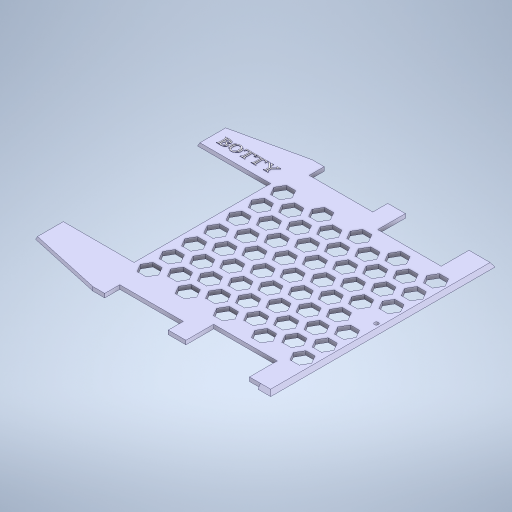
# Autodesk Inventor part: Bot v2 Top
Saved by Autodesk Inventor 2024 (Build 280153000, 153)
## iProperties
Created: 2023-11-01
Part Number: Bot v2 Top
Material: ABS Plastic
Document SubType Name: Modeling
Designer: CJ110
Density: 1.06 g/cm^3
Appearance: Smooth - White
Mass: 94.8046 g
Surface Area: 600.275 cm^2
Volume: 89.4383 cm^3
Author: CJ110
## iProperties of the stored document Bot v2 Top_3DPrint.ipt
Created: 2023-11-11
Part Number: Bot v2 Top_3DPrint
Material: Generic
Document SubType Name: Modeling
Designer: CJ110
Density: 1 g/cm^3
Appearance: Default
Author: CJ110
Autodesk Inventor part; units mm, degrees
(part 1 of 2)
ref_plane "YZ Plane" through (0, 0, 0) normal (1, 0, 0) x (0, 1, 0)
ref_plane "XZ Plane" through (0, 0, 0) normal (0, 1, 0) x (-1, 0, 0)
sketch "Sketch1" plane through (0, 0, 0) normal (0, 1, 0) x (-1, 0, 0)
  line L0 (0, 0) -> (144.1069, 0)
  line L1 (144.1069, 176.6621) -> (0, 176.6621)
  line L2 (0, 176.6621) -> (0, 0)
  line L3 (201.4652, 142.306) -> (144.8841, 142.306)
  line L4 (144.8841, 142.306) -> (144.8841, 34.356)
  line L5 (144.8841, 34.356) -> (201.4652, 34.356)
  line L6 (201.4652, 88.331) -> (0, 88.331) construction
  line L7 (144.1069, 176.6621) -> (201.4652, 164.0459)
  line L8 (201.4652, 12.6162) -> (144.1069, 0)
  line L9 (201.4652, 12.6162) -> (201.4652, 34.356)
  line L10 (201.4652, 142.306) -> (201.4652, 164.0459)
  line L11 (144.2491, 33.721) -> (144.2491, 142.941)
  line L12 (144.2491, 142.941) -> (200.8302, 142.941)
  line L13 (200.8302, 142.941) -> (200.8302, 163.5354)
  line L14 (200.8302, 163.5354) -> (144.0379, 176.0271)
  line L15 (144.0379, 176.0271) -> (0.635, 176.0271)
  line L16 (0.635, 176.0271) -> (0.635, 0.635)
  line L17 (0.635, 0.635) -> (144.0379, 0.635)
  line L18 (144.0379, 0.635) -> (200.8302, 13.1267)
  line L19 (200.8302, 13.1267) -> (200.8302, 33.721)
  line L20 (200.8302, 33.721) -> (144.2491, 33.721)
  line L21 (0.635, 176.0271) -> (0, 176.0271)
  line L22 (0.635, 0.635) -> (0, 0.635)
  point P0 (144.8841, 88.331)
  dimension "d0" = 176.6621
  dimension "d2" = 56.581
  dimension "d3" = 107.95
  dimension "d10" = 21.7399
  dimension "d11" = 144.1069
  dimension "d12" = 21.7399
  dimension "d52" = 201.4652
  dimension "d53" = 144.1069
  dimension "d54" = 0.635
  constraints: 46 end point, 12 perpendicular, 6 parallel, 3 horizontal, 3 point on line, 2 collinear, 2 midpoint, 9 other
  measures "d0" distance of L1.end L0.start
  measures "d2" distance of L3.start L3.end
  measures "d3" distance of L3.end L4.end
  measures "d10" distance from line of L7.end L3
  measures "d11" distance from line of L0.end L2
  measures "d12" distance from line of L8.start L5
  measures "d52" distance between parallel lines of L2 L9
  measures "d53" distance from line of L2 L1.start
  measures "d54" distance between parallel lines of L4 L11
extrude "Extrusion1" add sketch "Sketch1" along normal blind 3.175 contours L2 L21 L16 L22 | L16 L15 L14 L13 L12 L11 L20 L19 L18 L17
chamfer "Chamfer1" [suppressed]
sketch "Sketch2" plane through (0, 0, 0) normal (0, -1, 0) x (1, 0, 0)
  line L0 (0, 176.0271) -> (0, 0.635) projected
  line L1 (-145.8366, 33.721) -> (-145.8366, 142.941)
  line L2 (-144.0379, 176.0271) -> (0, 176.0271) projected
  line L3 (-200.8302, 163.5354) -> (-144.0379, 176.0271) projected
  line L4 (-200.8302, 142.941) -> (-200.8302, 163.5354) projected
  line L5 (-144.2491, 142.941) -> (-200.8302, 142.941) projected
  line L6 (-144.2491, 33.721) -> (-144.2491, 142.941) projected
  line L7 (-200.8302, 33.721) -> (-144.2491, 33.721) projected
  line L8 (-200.8302, 13.1267) -> (-200.8302, 33.721) projected
  line L9 (-144.0379, 0.635) -> (-200.8302, 13.1267) projected
  line L10 (0, 0.635) -> (-144.0379, 0.635) projected
  point P0 (0, 0)
  dimension "d55" = 1.5875
  constraints: 2 end point, 2 point on line
  measures "d55" distance between parallel lines of L6 L1
extrude "Extrusion2" add sketch "Sketch2" against normal blind 1.5875 contours L5 L6 L7 L1
sketch "Sketch3" plane through (0, 0, 195.7121) normal (1, 0, 0) x (0, 0, -1)
  line L0 (195.7121, 20.32) -> (195.7121, 0)
  line L1 (195.7121, 20.32) -> (183.0121, 20.32)
  line L2 (183.0121, 20.32) -> (195.7121, 0)
  line L3 (19.685, 0) -> (195.0771, 0) projected
  line L4 (19.685, 3.175) -> (195.0771, 3.175) projected
  line L5 (0, 0) -> (12.7, 20.32)
  line L6 (12.7, 20.32) -> (0, 20.32)
  line L7 (0, 20.32) -> (0, 0)
  line L8 (195.0771, 0) -> (195.0771, 3.175) projected
  line L9 (19.685, 0) -> (19.685, 3.175) projected
  point P0 (195.7121, 3.175)
  point P1 (193.7277, 3.175)
  point P2 (1.9844, 3.175)
  point P3 (195.0771, 1.016)
  point P4 (0.635, 1.016)
  dimension "d18" = 20.32
  dimension "d19" = 12.7
  dimension "d20" = 20.32
  dimension "d21" = 12.7
  constraints: 12 end point, 2 coincident, 2 horizontal, 2 vertical, 1 horizontal alignment
  measures "d18" distance of L0.start L0.end
  measures "d19" distance of L0.start L1.end
  measures "d20" distance of L6.end L5.start
  measures "d21" distance of L5.end L6.end
extrude "Extrusion3" [suppressed]
sketch "Sketch4" plane through (-147.1066, 0, 142.941) normal (0, 0, -1) x (-1, 0, 0)
  line L0 (53.7235, 0) -> (60.0735, 0)
  line L1 (53.7235, 0) -> (53.7235, 10.16)
  line L2 (53.7235, 10.16) -> (60.0735, 0)
  line L3 (53.7235, 0) -> (53.7235, 3.175) projected
  line L4 (-3.0688, 0) -> (53.7235, 0) projected
  line L5 (53.7235, 3.175) -> (55.7079, 0)
  point P0 (-147.1066, 0)
  point P1 (53.7235, 3.175)
  dimension "d38" = 6.35
  dimension "d39" = 10.16
  constraints: 8 end point, 2 collinear, 1 horizontal, 1 parallel, 1 point on line, 1 vertical
  measures "d38" distance of L0.start L0.end
  measures "d39" distance of L0.start L1.end
extrude "Extrusion4" add sketch "Sketch4" against normal up to surface contours L1 L5 L0 surface through (-200.8302, 0, 163.5354) normal (-0.2148189, 0, 0.9766539)
sketch "Sketch5" plane through (0, 3.175, 0) normal (0, 1, 0) x (1, 0, 0)
  line L0 (-144.1069, 0) -> (-201.4652, -22.1412) projected
  line L1 (-172.786, -11.0706) -> (-139.2855, -97.856)
  line L2 (-139.2855, -97.856) -> (-172.786, -184.6415)
  line L3 (-201.4652, -173.5709) -> (-144.1069, -195.7121) projected
  point P0 (0, 0)
  point P1 (-149.5475, -1.9844)
  point P2 (-199.4808, -23.2787)
  point P3 (-199.4808, -176.4009)
  point P4 (-149.5475, -197.6952)
  point P5 (-201.4652, -22.1412)
  point P6 (-144.1069, 0)
  point P7 (-146.116, -195.7121)
  constraints: 4 end point, 6 other
ref_plane "Work Plane1" through (-139.2855, 3.175, 97.856) normal (-0.9329073, 0, -0.3601166) x (-0.3601166, 0, 0.9329073)
ref_plane "Work Plane2" through (-172.786, 3.175, 11.0706) normal (-0.9329073, 0, 0.3601166) x (0.3601166, 0, 0.9329073)
sketch "Sketch6" plane through (-139.2855, 3.175, 97.856) normal (-0.9329073, 0, -0.3601166) x (-0.3601166, 0, 0.9329073)
  line L0 (82.1072, 17.145) -> (94.8072, -3.175)
  line L1 (94.8072, -3.175) -> (94.8072, 17.145)
  line L2 (94.8072, 17.145) -> (82.1072, 17.145)
  point P0 (-141.4496, -3.175)
  dimension "d30" = 12.7
  dimension "d31" = 20.32
  constraints: 6 end point, 1 coincident, 1 perpendicular, 1 vertical
  measures "d30" distance of L1.end L0.start
  measures "d31" distance of L0.end L1.end
extrude "Extrusion5" [suppressed]
sketch "Sketch7" plane through (-172.786, 3.175, 11.0706) normal (-0.9329073, 0, 0.3601166) x (0.3601166, 0, 0.9329073)
  line L0 (12.7, 17.145) -> (0, -3.175)
  line L1 (0, -3.175) -> (0, 17.145)
  line L2 (0, 17.145) -> (12.7, 17.145)
  point P0 (51.8953, -3.175)
  point P1 (0, -3.175)
  dimension "d34" = 12.7
  dimension "d35" = 20.32
  constraints: 6 end point, 1 coincident, 1 perpendicular, 1 vertical
  measures "d34" distance of L1.end L0.start
  measures "d35" distance of L0.end L1.end
extrude "Extrusion6" [suppressed]
ref_plane "Work Plane3" through (-144.2491, 1.5875, 88.331) normal (0, 0, -1) x (-1, 0, 0)
mirror "Mirror1" about plane through (-144.2491, 1.5875, 88.331) normal (0, 0, -1) of "Extrusion4"
sketch "Sketch8" plane through (0, 0, 176.6621) normal (1, 0, 0) x (0, 0, -1)
  line L0 (0.635, 0) -> (13.5632, 0) projected
  line L1 (0.635, 0) -> (-5.715, 0)
  line L2 (0.635, 0) -> (0.635, 10.16)
  line L3 (0.635, 10.16) -> (-5.715, 0)
  line L4 (0.635, 3.175) -> (-1.3494, 0)
  line L5 (0.635, 0) -> (0.635, 3.175) projected
  line L6 (0.635, 0) -> (176.0271, 0) projected
  line L7 (176.0271, 0) -> (176.0271, 3.175) projected
  line L8 (0.635, 3.175) -> (176.0271, 3.175) projected
  line L9 (0.635, 0) -> (0.635, 3.175) projected
  point P0 (176.6621, 0)
  point P1 (22.9072, 0)
  dimension "d40" = 6.35
  dimension "d41" = 10.16
  constraints: 8 end point, 2 collinear, 1 horizontal, 1 parallel, 1 point on line, 1 vertical
  measures "d40" distance of L0.start L1.end
  measures "d41" distance of L0.start L2.end
extrude "Extrusion7" add sketch "Sketch8" against normal blind 10.16 contours L1 L4 L2
mirror "Mirror2" about plane through (-144.2491, 1.5875, 88.331) normal (0, 0, -1) of "Extrusion7"
sketch "Sketch9" plane through (0, 3.175, 0) normal (0, 1, 0) x (1, 0, 0)
  line L0 (-69.6824, -175.4708) -> (-18.8824, -175.4708)
  line L1 (-18.8824, -175.4708) -> (-18.8824, -153.8808)
  line L2 (-18.8824, -153.8808) -> (-69.6824, -153.8808)
  line L3 (-69.6824, -153.8808) -> (-69.6824, -175.4708)
  line L4 (-134.5971, -175.4708) -> (-83.7971, -175.4708)
  line L5 (-83.7971, -175.4708) -> (-83.7971, -164.0408)
  line L6 (-83.7971, -164.0408) -> (-134.5971, -164.0408)
  line L7 (-134.5971, -164.0408) -> (-134.5971, -175.4708)
  line L8 (-144.2491, -33.721) -> (-144.2491, -142.941) projected
  line L9 (-144.2491, -88.331) -> (0, -88.331) construction
  line L10 (0, -176.0271) -> (0, -0.635) projected
  line L11 (-145.8366, -33.721) -> (-145.8366, -142.941) projected
  line L12 (-69.6824, -1.1913) -> (-18.8824, -1.1913)
  line L13 (-18.8824, -0.635) -> (-18.8824, -22.7813)
  line L14 (-18.8824, -22.7813) -> (-69.6824, -22.7813)
  line L15 (-69.6824, -22.7813) -> (-69.6824, -0.635)
  line L16 (-134.5971, -1.1913) -> (-83.7971, -1.1913)
  line L17 (-83.7971, -0.635) -> (-83.7971, -12.6213)
  line L18 (-83.7971, -12.6213) -> (-134.5971, -12.6213)
  line L19 (-134.5971, -12.6213) -> (-134.5971, -0.635)
  line L20 (0, -0.635) -> (0, -176.0271)
  line L21 (-69.6824, -175.4708) -> (-69.6824, -176.0271)
  line L22 (-144.0379, -176.0271) -> (-10.16, -176.0271) projected
  line L23 (-18.8824, -175.4708) -> (-18.8824, -176.0271)
  line L24 (-83.7971, -175.4708) -> (-83.7971, -176.0271)
  line L25 (-134.5971, -175.4708) -> (-134.5971, -176.0271)
  line L26 (0, -176.0271) -> (0, -0.635) projected
  line L27 (0, -0.635) -> (-10.16, -0.635) projected
  line L28 (-10.16, -0.635) -> (-144.0379, -0.635) projected
  line L29 (-144.0379, -0.635) -> (-200.8302, -13.1267) projected
  line L30 (-200.8302, -13.1267) -> (-200.8302, -33.721) projected
  line L31 (-200.8302, -33.721) -> (-144.2491, -33.721) projected
  line L32 (-144.2491, -33.721) -> (-144.2491, -142.941) projected
  line L33 (-144.2491, -142.941) -> (-200.8302, -142.941) projected
  line L34 (-200.8302, -142.941) -> (-200.8302, -163.5354) projected
  line L35 (-200.8302, -163.5354) -> (-144.0379, -176.0271) projected
  line L36 (-144.0379, -176.0271) -> (-10.16, -176.0271) projected
  line L37 (-10.16, -176.0271) -> (0, -176.0271) projected
  point P0 (0, 0)
  point P1 (-44.2824, -153.8808)
  point P2 (-109.1971, -164.0408)
  point P3 (-44.2824, -22.7813)
  point P4 (-109.1971, -12.6213)
  point P5 (-83.7971, -176.0271)
  point P6 (-18.8824, -176.0271)
  dimension "d44" = 11.43
  dimension "d45" = 21.59
  dimension "d60" = 65.5498
  dimension "d61" = 50.8
  dimension "d62" = 50.8
  dimension "d63" = 64.9148
  dimension "d69" = 9.652
  constraints: 44 end point, 14 point on line, 12 symmetric about line, 5 perpendicular, 4 midpoint, 4 parallel, 2 horizontal, 1 vertical
  measures "d44" distance between parallel lines of L6 L4
  measures "d45" distance between parallel lines of L2 L0
  measures "d60" distance between parallel lines of L9 L2
  measures "d61" distance between parallel lines of L7 L5
  measures "d62" distance of L1.end L2.end
  measures "d63" horizontal distance of point (-44.282, -153.881) point (-109.197, -164.041)
  measures "d69" distance between parallel lines of L7 L8
sketch "Sketch11" plane through (-144.2491, 1.5875, 88.331) normal (0, 0, -1) x (-1, 0, 0)
  line L0 (-144.2491, 1.5875) -> (-144.2491, -1.5875) projected
  line L1 (-144.2491, -1.5875) -> (-150.5991, -1.5875)
  line L2 (-150.5991, -1.5875) -> (-144.2491, 8.5725)
  line L3 (-144.2491, 8.5725) -> (-144.2491, -1.5875)
  line L4 (-144.2491, -1.5875) -> (-142.2648, 1.5875)
  line L5 (-134.0891, 1.5875) -> (-144.2491, 1.5875) projected
  dimension "d56" = 6.35
  dimension "d57" = 10.16
  constraints: 8 end point, 1 horizontal, 1 parallel, 1 perpendicular, 1 point on line
  measures "d56" distance of L0.end L1.end
  measures "d57" distance of L2.end L0.end
extrude "Extrusion9" cut sketch "Sketch11" along normal through all both and the other way through all contours L5 L4 L0
extrude "Extrusion10" cut sketch "Sketch9" against normal through all contours L3 L2 L1 L0 | L0 L23 L22 L21 | L22 L25 L4 L24 | L4 L7 L6 L5 | L13 L12 L15 L28 | L13 L14 L15 L12 | L17 L16 L19 L28 | L17 L18 L19 L16
sketch "Sketch12" plane through (0, 3.175, 0) normal (0, 1, 0) x (1, 0, 0)
  line L0 (-1.9844, -176.0271) -> (-1.9844, -0.635) projected
  line L1 (-1.9844, -88.331) -> (-144.2491, -88.331) construction
  line L2 (-144.2491, -33.721) -> (-144.2491, -142.941) projected
  circle A0 centre (-5.1594, -88.331) radius 1.5875
  point P0 (0, 0)
  dimension "d70" = 3.175
  dimension "d71" = 3.175
  constraints: 2 end point, 2 midpoint, 1 centre point, 1 point on line
  measures "d70" diameter of A0
  measures "d71" distance from line of L0 A0.centre
extrude "Extrusion11" cut sketch "Sketch12" against normal through all
sketch "Sketch16" plane through (0, 3.175, 0) normal (0, 1, 0) x (1, 0, 0)
  line L0 (-140.4391, -141.671) -> (-136.773, -135.321)
  line L1 (-136.773, -135.321) -> (-129.4406, -135.321)
  line L2 (-129.4406, -135.321) -> (-125.7744, -141.671)
  line L3 (-125.7744, -141.671) -> (-129.4406, -148.021)
  line L4 (-129.4406, -148.021) -> (-136.773, -148.021)
  line L5 (-136.773, -148.021) -> (-140.4391, -141.671)
  line L6 (-125.0412, -132.781) -> (-121.375, -126.431)
  line L7 (-121.375, -126.431) -> (-114.0427, -126.431)
  line L8 (-114.0427, -126.431) -> (-110.3765, -132.781)
  line L9 (-110.3765, -132.781) -> (-114.0427, -139.131)
  line L10 (-114.0427, -139.131) -> (-121.375, -139.131)
  line L11 (-121.375, -139.131) -> (-125.0412, -132.781)
  line L12 (-140.4391, -123.891) -> (-136.773, -117.541)
  line L13 (-136.773, -117.541) -> (-129.4406, -117.541)
  line L14 (-129.4406, -117.541) -> (-125.7744, -123.891)
  line L15 (-125.7744, -123.891) -> (-129.4406, -130.241)
  line L16 (-129.4406, -130.241) -> (-136.773, -130.241)
  line L17 (-136.773, -130.241) -> (-140.4391, -123.891)
  line L18 (-125.0412, -115.001) -> (-121.375, -108.651)
  line L19 (-121.375, -108.651) -> (-114.0427, -108.651)
  line L20 (-114.0427, -108.651) -> (-110.3765, -115.001)
  line L21 (-110.3765, -115.001) -> (-114.0427, -121.351)
  line L22 (-114.0427, -121.351) -> (-121.375, -121.351)
  line L23 (-121.375, -121.351) -> (-125.0412, -115.001)
  circle A0 centre (-5.1594, -97.856) radius 1.5875 projected
  line L24 (-69.6824, -22.7813) -> (-69.6824, -0.635) projected
  line L25 (-69.6824, -0.635) -> (-83.7971, -0.635) projected
  line L26 (-83.7971, -0.635) -> (-83.7971, -12.6213) projected
  line L27 (-83.7971, -12.6213) -> (-134.5971, -12.6213) projected
  line L28 (-134.5971, -12.6213) -> (-134.5971, -0.635) projected
  line L29 (-134.5971, -0.635) -> (-143.9886, -0.635) projected
  line L30 (-143.9886, -0.635) -> (-200.8302, -22.5767) projected
  line L31 (-200.8302, -22.5767) -> (-200.8302, -43.246) projected
  line L32 (-200.8302, -43.246) -> (-144.2491, -43.246) projected
  line L33 (-144.2491, -43.246) -> (-144.2491, -152.466) projected
  line L34 (-144.2491, -152.466) -> (-200.8302, -152.466) projected
  line L35 (-200.8302, -152.466) -> (-200.8302, -173.1354) projected
  line L36 (-200.8302, -173.1354) -> (-143.9886, -195.0771) projected
  line L37 (-143.9886, -195.0771) -> (-134.5971, -195.0771) projected
  line L38 (-134.5971, -195.0771) -> (-134.5971, -183.0908) projected
  line L39 (-134.5971, -183.0908) -> (-83.7971, -183.0908) projected
  line L40 (-83.7971, -183.0908) -> (-83.7971, -195.0771) projected
  line L41 (-83.7971, -195.0771) -> (-69.6824, -195.0771) projected
  line L42 (-69.6824, -195.0771) -> (-69.6824, -172.9308) projected
  line L43 (-69.6824, -172.9308) -> (-18.8824, -172.9308) projected
  line L44 (-18.8824, -172.9308) -> (-18.8824, -195.0771) projected
  line L45 (-18.8824, -195.0771) -> (-10.16, -195.0771) projected
  line L46 (-10.16, -195.0771) -> (-1.9844, -195.0771) projected
  line L47 (-1.9844, -195.0771) -> (-1.9844, -0.635) projected
  line L48 (-1.9844, -0.635) -> (-10.16, -0.635) projected
  line L49 (-10.16, -0.635) -> (-18.8824, -0.635) projected
  line L50 (-18.8824, -0.635) -> (-18.8824, -22.7813) projected
  line L51 (-18.8824, -22.7813) -> (-69.6824, -22.7813) projected
  line L52 (-110.3765, -97.221) -> (-114.0427, -103.571)
  line L53 (-114.0427, -73.091) -> (-110.3765, -79.441)
  line L54 (-114.0427, -90.871) -> (-110.3765, -97.221)
  line L55 (-125.7744, -106.111) -> (-129.4406, -112.461)
  line L56 (-129.4406, -99.761) -> (-125.7744, -106.111)
  line L57 (-121.375, -73.091) -> (-114.0427, -73.091)
  line L58 (-129.4406, -112.461) -> (-136.773, -112.461)
  line L59 (-136.773, -112.461) -> (-140.4391, -106.111)
  line L60 (-125.0412, -79.441) -> (-121.375, -73.091)
  line L61 (-140.4391, -106.111) -> (-136.773, -99.761)
  line L62 (-121.375, -103.571) -> (-125.0412, -97.221)
  line L63 (-114.0427, -103.571) -> (-121.375, -103.571)
  line L64 (-125.0412, -97.221) -> (-121.375, -90.871)
  line L65 (-121.375, -90.871) -> (-114.0427, -90.871)
  line L66 (-136.773, -99.761) -> (-129.4406, -99.761)
  line L67 (-114.0427, -85.791) -> (-121.375, -85.791)
  line L68 (-110.3765, -79.441) -> (-114.0427, -85.791)
  line L69 (-121.375, -85.791) -> (-125.0412, -79.441)
  line L70 (-129.4406, -94.681) -> (-136.773, -94.681)
  line L71 (-129.4406, -81.981) -> (-125.7744, -88.331)
  line L72 (-136.773, -94.681) -> (-140.4391, -88.331)
  line L73 (-136.773, -81.981) -> (-129.4406, -81.981)
  line L74 (-140.4391, -88.331) -> (-136.773, -81.981)
  line L75 (-125.7744, -88.331) -> (-129.4406, -94.681)
  line L76 (-110.3765, -61.661) -> (-114.0427, -68.011)
  line L77 (-114.0427, -37.531) -> (-110.3765, -43.881)
  line L78 (-114.0427, -55.311) -> (-110.3765, -61.661)
  line L79 (-125.7744, -70.551) -> (-129.4406, -76.901)
  line L80 (-129.4406, -64.201) -> (-125.7744, -70.551)
  line L81 (-121.375, -37.531) -> (-114.0427, -37.531)
  line L82 (-129.4406, -76.901) -> (-136.773, -76.901)
  line L83 (-136.773, -76.901) -> (-140.4391, -70.551)
  line L84 (-125.0412, -43.881) -> (-121.375, -37.531)
  line L85 (-140.4391, -70.551) -> (-136.773, -64.201)
  line L86 (-121.375, -68.011) -> (-125.0412, -61.661)
  line L87 (-114.0427, -68.011) -> (-121.375, -68.011)
  line L88 (-125.0412, -61.661) -> (-121.375, -55.311)
  line L89 (-121.375, -55.311) -> (-114.0427, -55.311)
  line L90 (-136.773, -64.201) -> (-129.4406, -64.201)
  line L91 (-114.0427, -50.231) -> (-121.375, -50.231)
  line L92 (-110.3765, -43.881) -> (-114.0427, -50.231)
  line L93 (-121.375, -50.231) -> (-125.0412, -43.881)
  line L94 (-129.4406, -59.121) -> (-136.773, -59.121)
  line L95 (-129.4406, -46.421) -> (-125.7744, -52.771)
  line L96 (-136.773, -59.121) -> (-140.4391, -52.771)
  line L97 (-136.773, -46.421) -> (-129.4406, -46.421)
  line L98 (-140.4391, -52.771) -> (-136.773, -46.421)
  line L99 (-125.7744, -52.771) -> (-129.4406, -59.121)
  line L100 (-79.8965, -132.781) -> (-83.5627, -139.131)
  line L101 (-83.5627, -108.651) -> (-79.8965, -115.001)
  line L102 (-83.5627, -126.431) -> (-79.8965, -132.781)
  line L103 (-95.2944, -141.671) -> (-98.9606, -148.021)
  line L104 (-98.9606, -135.321) -> (-95.2944, -141.671)
  line L105 (-90.895, -108.651) -> (-83.5627, -108.651)
  line L106 (-98.9606, -148.021) -> (-106.293, -148.021)
  line L107 (-106.293, -148.021) -> (-109.9591, -141.671)
  line L108 (-94.5612, -115.001) -> (-90.895, -108.651)
  line L109 (-109.9591, -141.671) -> (-106.293, -135.321)
  line L110 (-90.895, -139.131) -> (-94.5612, -132.781)
  line L111 (-83.5627, -139.131) -> (-90.895, -139.131)
  line L112 (-94.5612, -132.781) -> (-90.895, -126.431)
  line L113 (-90.895, -126.431) -> (-83.5627, -126.431)
  line L114 (-106.293, -135.321) -> (-98.9606, -135.321)
  line L115 (-83.5627, -121.351) -> (-90.895, -121.351)
  line L116 (-79.8965, -115.001) -> (-83.5627, -121.351)
  line L117 (-90.895, -121.351) -> (-94.5612, -115.001)
  line L118 (-98.9606, -130.241) -> (-106.293, -130.241)
  line L119 (-98.9606, -117.541) -> (-95.2944, -123.891)
  line L120 (-106.293, -130.241) -> (-109.9591, -123.891)
  line L121 (-106.293, -117.541) -> (-98.9606, -117.541)
  line L122 (-109.9591, -123.891) -> (-106.293, -117.541)
  line L123 (-95.2944, -123.891) -> (-98.9606, -130.241)
  line L124 (-79.8965, -97.221) -> (-83.5627, -103.571)
  line L125 (-83.5627, -73.091) -> (-79.8965, -79.441)
  line L126 (-83.5627, -90.871) -> (-79.8965, -97.221)
  line L127 (-95.2944, -106.111) -> (-98.9606, -112.461)
  line L128 (-98.9606, -99.761) -> (-95.2944, -106.111)
  line L129 (-90.895, -73.091) -> (-83.5627, -73.091)
  line L130 (-98.9606, -112.461) -> (-106.293, -112.461)
  line L131 (-106.293, -112.461) -> (-109.9591, -106.111)
  line L132 (-94.5612, -79.441) -> (-90.895, -73.091)
  line L133 (-109.9591, -106.111) -> (-106.293, -99.761)
  line L134 (-90.895, -103.571) -> (-94.5612, -97.221)
  line L135 (-83.5627, -103.571) -> (-90.895, -103.571)
  line L136 (-94.5612, -97.221) -> (-90.895, -90.871)
  line L137 (-90.895, -90.871) -> (-83.5627, -90.871)
  line L138 (-106.293, -99.761) -> (-98.9606, -99.761)
  line L139 (-83.5627, -85.791) -> (-90.895, -85.791)
  line L140 (-79.8965, -79.441) -> (-83.5627, -85.791)
  line L141 (-90.895, -85.791) -> (-94.5612, -79.441)
  line L142 (-98.9606, -94.681) -> (-106.293, -94.681)
  line L143 (-98.9606, -81.981) -> (-95.2944, -88.331)
  line L144 (-106.293, -94.681) -> (-109.9591, -88.331)
  line L145 (-106.293, -81.981) -> (-98.9606, -81.981)
  line L146 (-109.9591, -88.331) -> (-106.293, -81.981)
  line L147 (-95.2944, -88.331) -> (-98.9606, -94.681)
  line L148 (-79.8965, -61.661) -> (-83.5627, -68.011)
  line L149 (-83.5627, -37.531) -> (-79.8965, -43.881)
  line L150 (-83.5627, -55.311) -> (-79.8965, -61.661)
  line L151 (-95.2944, -70.551) -> (-98.9606, -76.901)
  line L152 (-98.9606, -64.201) -> (-95.2944, -70.551)
  line L153 (-90.895, -37.531) -> (-83.5627, -37.531)
  line L154 (-98.9606, -76.901) -> (-106.293, -76.901)
  line L155 (-106.293, -76.901) -> (-109.9591, -70.551)
  line L156 (-94.5612, -43.881) -> (-90.895, -37.531)
  line L157 (-109.9591, -70.551) -> (-106.293, -64.201)
  line L158 (-90.895, -68.011) -> (-94.5612, -61.661)
  line L159 (-83.5627, -68.011) -> (-90.895, -68.011)
  line L160 (-94.5612, -61.661) -> (-90.895, -55.311)
  line L161 (-90.895, -55.311) -> (-83.5627, -55.311)
  line L162 (-106.293, -64.201) -> (-98.9606, -64.201)
  line L163 (-83.5627, -50.231) -> (-90.895, -50.231)
  line L164 (-79.8965, -43.881) -> (-83.5627, -50.231)
  line L165 (-90.895, -50.231) -> (-94.5612, -43.881)
  line L166 (-98.9606, -59.121) -> (-106.293, -59.121)
  line L167 (-98.9606, -46.421) -> (-95.2944, -52.771)
  line L168 (-106.293, -59.121) -> (-109.9591, -52.771)
  line L169 (-106.293, -46.421) -> (-98.9606, -46.421)
  line L170 (-109.9591, -52.771) -> (-106.293, -46.421)
  line L171 (-95.2944, -52.771) -> (-98.9606, -59.121)
  line L172 (-49.4165, -132.781) -> (-53.0827, -139.131)
  line L173 (-53.0827, -108.651) -> (-49.4165, -115.001)
  line L174 (-53.0827, -126.431) -> (-49.4165, -132.781)
  line L175 (-64.8144, -141.671) -> (-68.4806, -148.021)
  line L176 (-68.4806, -135.321) -> (-64.8144, -141.671)
  line L177 (-60.415, -108.651) -> (-53.0827, -108.651)
  line L178 (-68.4806, -148.021) -> (-75.813, -148.021)
  line L179 (-75.813, -148.021) -> (-79.4791, -141.671)
  line L180 (-64.0812, -115.001) -> (-60.415, -108.651)
  line L181 (-79.4791, -141.671) -> (-75.813, -135.321)
  line L182 (-60.415, -139.131) -> (-64.0812, -132.781)
  line L183 (-53.0827, -139.131) -> (-60.415, -139.131)
  line L184 (-64.0812, -132.781) -> (-60.415, -126.431)
  line L185 (-60.415, -126.431) -> (-53.0827, -126.431)
  line L186 (-75.813, -135.321) -> (-68.4806, -135.321)
  line L187 (-53.0827, -121.351) -> (-60.415, -121.351)
  line L188 (-49.4165, -115.001) -> (-53.0827, -121.351)
  line L189 (-60.415, -121.351) -> (-64.0812, -115.001)
  line L190 (-68.4806, -130.241) -> (-75.813, -130.241)
  line L191 (-68.4806, -117.541) -> (-64.8144, -123.891)
  line L192 (-75.813, -130.241) -> (-79.4791, -123.891)
  line L193 (-75.813, -117.541) -> (-68.4806, -117.541)
  line L194 (-79.4791, -123.891) -> (-75.813, -117.541)
  line L195 (-64.8144, -123.891) -> (-68.4806, -130.241)
  line L196 (-49.4165, -97.221) -> (-53.0827, -103.571)
  line L197 (-53.0827, -73.091) -> (-49.4165, -79.441)
  line L198 (-53.0827, -90.871) -> (-49.4165, -97.221)
  line L199 (-64.8144, -106.111) -> (-68.4806, -112.461)
  line L200 (-68.4806, -99.761) -> (-64.8144, -106.111)
  line L201 (-60.415, -73.091) -> (-53.0827, -73.091)
  line L202 (-68.4806, -112.461) -> (-75.813, -112.461)
  line L203 (-75.813, -112.461) -> (-79.4791, -106.111)
  line L204 (-64.0812, -79.441) -> (-60.415, -73.091)
  line L205 (-79.4791, -106.111) -> (-75.813, -99.761)
  line L206 (-60.415, -103.571) -> (-64.0812, -97.221)
  line L207 (-53.0827, -103.571) -> (-60.415, -103.571)
  line L208 (-64.0812, -97.221) -> (-60.415, -90.871)
  line L209 (-60.415, -90.871) -> (-53.0827, -90.871)
  line L210 (-75.813, -99.761) -> (-68.4806, -99.761)
  line L211 (-53.0827, -85.791) -> (-60.415, -85.791)
  line L212 (-49.4165, -79.441) -> (-53.0827, -85.791)
  line L213 (-60.415, -85.791) -> (-64.0812, -79.441)
  line L214 (-68.4806, -94.681) -> (-75.813, -94.681)
  line L215 (-68.4806, -81.981) -> (-64.8144, -88.331)
  line L216 (-75.813, -94.681) -> (-79.4791, -88.331)
  line L217 (-75.813, -81.981) -> (-68.4806, -81.981)
  line L218 (-79.4791, -88.331) -> (-75.813, -81.981)
  line L219 (-64.8144, -88.331) -> (-68.4806, -94.681)
  line L220 (-49.4165, -61.661) -> (-53.0827, -68.011)
  line L221 (-53.0827, -37.531) -> (-49.4165, -43.881)
  line L222 (-53.0827, -55.311) -> (-49.4165, -61.661)
  line L223 (-64.8144, -70.551) -> (-68.4806, -76.901)
  line L224 (-68.4806, -64.201) -> (-64.8144, -70.551)
  line L225 (-60.415, -37.531) -> (-53.0827, -37.531)
  line L226 (-68.4806, -76.901) -> (-75.813, -76.901)
  line L227 (-75.813, -76.901) -> (-79.4791, -70.551)
  line L228 (-64.0812, -43.881) -> (-60.415, -37.531)
  line L229 (-79.4791, -70.551) -> (-75.813, -64.201)
  line L230 (-60.415, -68.011) -> (-64.0812, -61.661)
  line L231 (-53.0827, -68.011) -> (-60.415, -68.011)
  line L232 (-64.0812, -61.661) -> (-60.415, -55.311)
  line L233 (-60.415, -55.311) -> (-53.0827, -55.311)
  line L234 (-75.813, -64.201) -> (-68.4806, -64.201)
  line L235 (-53.0827, -50.231) -> (-60.415, -50.231)
  line L236 (-49.4165, -43.881) -> (-53.0827, -50.231)
  line L237 (-60.415, -50.231) -> (-64.0812, -43.881)
  line L238 (-68.4806, -59.121) -> (-75.813, -59.121)
  line L239 (-68.4806, -46.421) -> (-64.8144, -52.771)
  line L240 (-75.813, -59.121) -> (-79.4791, -52.771)
  line L241 (-75.813, -46.421) -> (-68.4806, -46.421)
  line L242 (-79.4791, -52.771) -> (-75.813, -46.421)
  line L243 (-64.8144, -52.771) -> (-68.4806, -59.121)
  line L244 (-18.9365, -132.781) -> (-22.6027, -139.131)
  line L245 (-22.6027, -108.651) -> (-18.9365, -115.001)
  line L246 (-22.6027, -126.431) -> (-18.9365, -132.781)
  line L247 (-34.3344, -141.671) -> (-38.0006, -148.021)
  line L248 (-38.0006, -135.321) -> (-34.3344, -141.671)
  line L249 (-29.935, -108.651) -> (-22.6027, -108.651)
  line L250 (-38.0006, -148.021) -> (-45.333, -148.021)
  line L251 (-45.333, -148.021) -> (-48.9991, -141.671)
  line L252 (-33.6012, -115.001) -> (-29.935, -108.651)
  line L253 (-48.9991, -141.671) -> (-45.333, -135.321)
  line L254 (-29.935, -139.131) -> (-33.6012, -132.781)
  line L255 (-22.6027, -139.131) -> (-29.935, -139.131)
  line L256 (-33.6012, -132.781) -> (-29.935, -126.431)
  line L257 (-29.935, -126.431) -> (-22.6027, -126.431)
  line L258 (-45.333, -135.321) -> (-38.0006, -135.321)
  line L259 (-22.6027, -121.351) -> (-29.935, -121.351)
  line L260 (-18.9365, -115.001) -> (-22.6027, -121.351)
  line L261 (-29.935, -121.351) -> (-33.6012, -115.001)
  line L262 (-38.0006, -130.241) -> (-45.333, -130.241)
  line L263 (-38.0006, -117.541) -> (-34.3344, -123.891)
  line L264 (-45.333, -130.241) -> (-48.9991, -123.891)
  line L265 (-45.333, -117.541) -> (-38.0006, -117.541)
  line L266 (-48.9991, -123.891) -> (-45.333, -117.541)
  line L267 (-34.3344, -123.891) -> (-38.0006, -130.241)
  line L268 (-18.9365, -97.221) -> (-22.6027, -103.571)
  line L269 (-22.6027, -73.091) -> (-18.9365, -79.441)
  line L270 (-22.6027, -90.871) -> (-18.9365, -97.221)
  line L271 (-34.3344, -106.111) -> (-38.0006, -112.461)
  line L272 (-38.0006, -99.761) -> (-34.3344, -106.111)
  line L273 (-29.935, -73.091) -> (-22.6027, -73.091)
  line L274 (-38.0006, -112.461) -> (-45.333, -112.461)
  line L275 (-45.333, -112.461) -> (-48.9991, -106.111)
  line L276 (-33.6012, -79.441) -> (-29.935, -73.091)
  line L277 (-48.9991, -106.111) -> (-45.333, -99.761)
  line L278 (-29.935, -103.571) -> (-33.6012, -97.221)
  line L279 (-22.6027, -103.571) -> (-29.935, -103.571)
  line L280 (-33.6012, -97.221) -> (-29.935, -90.871)
  line L281 (-29.935, -90.871) -> (-22.6027, -90.871)
  line L282 (-45.333, -99.761) -> (-38.0006, -99.761)
  line L283 (-22.6027, -85.791) -> (-29.935, -85.791)
  line L284 (-18.9365, -79.441) -> (-22.6027, -85.791)
  line L285 (-29.935, -85.791) -> (-33.6012, -79.441)
  line L286 (-38.0006, -94.681) -> (-45.333, -94.681)
  line L287 (-38.0006, -81.981) -> (-34.3344, -88.331)
  line L288 (-45.333, -94.681) -> (-48.9991, -88.331)
  line L289 (-45.333, -81.981) -> (-38.0006, -81.981)
  line L290 (-48.9991, -88.331) -> (-45.333, -81.981)
  line L291 (-34.3344, -88.331) -> (-38.0006, -94.681)
  line L292 (-18.9365, -61.661) -> (-22.6027, -68.011)
  line L293 (-22.6027, -37.531) -> (-18.9365, -43.881)
  line L294 (-22.6027, -55.311) -> (-18.9365, -61.661)
  line L295 (-34.3344, -70.551) -> (-38.0006, -76.901)
  line L296 (-38.0006, -64.201) -> (-34.3344, -70.551)
  line L297 (-29.935, -37.531) -> (-22.6027, -37.531)
  line L298 (-38.0006, -76.901) -> (-45.333, -76.901)
  line L299 (-45.333, -76.901) -> (-48.9991, -70.551)
  line L300 (-33.6012, -43.881) -> (-29.935, -37.531)
  line L301 (-48.9991, -70.551) -> (-45.333, -64.201)
  line L302 (-29.935, -68.011) -> (-33.6012, -61.661)
  line L303 (-22.6027, -68.011) -> (-29.935, -68.011)
  line L304 (-33.6012, -61.661) -> (-29.935, -55.311)
  line L305 (-29.935, -55.311) -> (-22.6027, -55.311)
  line L306 (-45.333, -64.201) -> (-38.0006, -64.201)
  line L307 (-22.6027, -50.231) -> (-29.935, -50.231)
  line L308 (-18.9365, -43.881) -> (-22.6027, -50.231)
  line L309 (-29.935, -50.231) -> (-33.6012, -43.881)
  line L310 (-38.0006, -59.121) -> (-45.333, -59.121)
  line L311 (-38.0006, -46.421) -> (-34.3344, -52.771)
  line L312 (-45.333, -59.121) -> (-48.9991, -52.771)
  line L313 (-45.333, -46.421) -> (-38.0006, -46.421)
  line L314 (-48.9991, -52.771) -> (-45.333, -46.421)
  line L315 (-34.3344, -52.771) -> (-38.0006, -59.121)
  line L316 (-140.4391, -34.991) -> (-136.773, -28.641)
  line L317 (-136.773, -28.641) -> (-129.4406, -28.641)
  line L318 (-129.4406, -28.641) -> (-125.7744, -34.991)
  line L319 (-125.7744, -34.991) -> (-129.4406, -41.341)
  line L320 (-129.4406, -41.341) -> (-136.773, -41.341)
  line L321 (-136.773, -41.341) -> (-140.4391, -34.991)
  line L322 (-109.9591, -34.991) -> (-106.293, -28.641)
  line L323 (-106.293, -28.641) -> (-98.9606, -28.641)
  line L324 (-98.9606, -28.641) -> (-95.2944, -34.991)
  line L325 (-95.2944, -34.991) -> (-98.9606, -41.341)
  line L326 (-98.9606, -41.341) -> (-106.293, -41.341)
  line L327 (-106.293, -41.341) -> (-109.9591, -34.991)
  line L328 (-79.4791, -34.991) -> (-75.813, -28.641)
  line L329 (-75.813, -28.641) -> (-68.4806, -28.641)
  line L330 (-68.4806, -28.641) -> (-64.8144, -34.991)
  line L331 (-64.8144, -34.991) -> (-68.4806, -41.341)
  line L332 (-68.4806, -41.341) -> (-75.813, -41.341)
  line L333 (-75.813, -41.341) -> (-79.4791, -34.991)
  line L334 (-48.9991, -34.991) -> (-45.333, -28.641)
  line L335 (-45.333, -28.641) -> (-38.0006, -28.641)
  line L336 (-38.0006, -28.641) -> (-34.3344, -34.991)
  line L337 (-34.3344, -34.991) -> (-38.0006, -41.341)
  line L338 (-38.0006, -41.341) -> (-45.333, -41.341)
  line L339 (-45.333, -41.341) -> (-48.9991, -34.991)
  line L340 (-18.2033, -141.671) -> (-14.5371, -135.321)
  line L341 (-14.5371, -135.321) -> (-7.2048, -135.321)
  line L342 (-7.2048, -135.321) -> (-3.5386, -141.671)
  line L343 (-3.5386, -141.671) -> (-7.2048, -148.021)
  line L344 (-7.2048, -148.021) -> (-14.5371, -148.021)
  line L345 (-14.5371, -148.021) -> (-18.2033, -141.671)
  line L346 (-18.2033, -123.891) -> (-14.5371, -117.541)
  line L347 (-14.5371, -117.541) -> (-7.2048, -117.541)
  line L348 (-7.2048, -117.541) -> (-3.5386, -123.891)
  line L349 (-3.5386, -123.891) -> (-7.2048, -130.241)
  line L350 (-7.2048, -130.241) -> (-14.5371, -130.241)
  line L351 (-14.5371, -130.241) -> (-18.2033, -123.891)
  line L352 (-18.2033, -106.111) -> (-14.5371, -99.761)
  line L353 (-14.5371, -99.761) -> (-7.2048, -99.761)
  line L354 (-7.2048, -99.761) -> (-3.5386, -106.111)
  line L355 (-3.5386, -106.111) -> (-7.2048, -112.461)
  line L356 (-7.2048, -112.461) -> (-14.5371, -112.461)
  line L357 (-14.5371, -112.461) -> (-18.2033, -106.111)
  line L358 (-18.2033, -70.551) -> (-14.5371, -64.201)
  line L359 (-14.5371, -64.201) -> (-7.2048, -64.201)
  line L360 (-7.2048, -64.201) -> (-3.5386, -70.551)
  line L361 (-3.5386, -70.551) -> (-7.2048, -76.901)
  line L362 (-7.2048, -76.901) -> (-14.5371, -76.901)
  line L363 (-14.5371, -76.901) -> (-18.2033, -70.551)
  line L364 (-18.2033, -52.771) -> (-14.5371, -46.421)
  line L365 (-14.5371, -46.421) -> (-7.2048, -46.421)
  line L366 (-7.2048, -46.421) -> (-3.5386, -52.771)
  line L367 (-3.5386, -52.771) -> (-7.2048, -59.121)
  line L368 (-7.2048, -59.121) -> (-14.5371, -59.121)
  line L369 (-14.5371, -59.121) -> (-18.2033, -52.771)
  line L370 (-18.2033, -34.991) -> (-14.5371, -28.641)
  line L371 (-14.5371, -28.641) -> (-7.2048, -28.641)
  line L372 (-7.2048, -28.641) -> (-3.5386, -34.991)
  line L373 (-3.5386, -34.991) -> (-7.2048, -41.341)
  line L374 (-7.2048, -41.341) -> (-14.5371, -41.341)
  line L375 (-14.5371, -41.341) -> (-18.2033, -34.991)
  circle A1 centre (-5.1594, -88.331) radius 1.5875 projected
  line L376 (-83.7971, -164.0408) -> (-83.7971, -176.0271) projected
  line L377 (-83.7971, -176.0271) -> (-69.6824, -176.0271) projected
  line L378 (-69.6824, -176.0271) -> (-69.6824, -153.8808) projected
  line L379 (-69.6824, -153.8808) -> (-18.8824, -153.8808) projected
  line L380 (-18.8824, -153.8808) -> (-18.8824, -176.0271) projected
  line L381 (-18.8824, -176.0271) -> (-10.16, -176.0271) projected
  line L382 (-10.16, -176.0271) -> (-1.9844, -176.0271) projected
  line L383 (-1.9844, -176.0271) -> (-1.9844, -0.635) projected
  line L384 (-1.9844, -0.635) -> (-10.16, -0.635) projected
  line L385 (-10.16, -0.635) -> (-18.8824, -0.635) projected
  line L386 (-18.8824, -0.635) -> (-18.8824, -22.7813) projected
  line L387 (-18.8824, -22.7813) -> (-69.6824, -22.7813) projected
  line L388 (-69.6824, -22.7813) -> (-69.6824, -0.635) projected
  line L389 (-69.6824, -0.635) -> (-83.7971, -0.635) projected
  line L390 (-83.7971, -0.635) -> (-83.7971, -12.6213) projected
  line L391 (-83.7971, -12.6213) -> (-134.5971, -12.6213) projected
  line L392 (-134.5971, -12.6213) -> (-134.5971, -0.635) projected
  line L393 (-134.5971, -0.635) -> (-144.0379, -0.635) projected
  line L394 (-144.0379, -0.635) -> (-200.8302, -13.1267) projected
  line L395 (-200.8302, -13.1267) -> (-200.8302, -33.721) projected
  line L396 (-200.8302, -33.721) -> (-144.2491, -33.721) projected
  line L397 (-144.2491, -33.721) -> (-144.2491, -142.941) projected
  line L398 (-144.2491, -142.941) -> (-200.8302, -142.941) projected
  line L399 (-200.8302, -142.941) -> (-200.8302, -163.5354) projected
  line L400 (-200.8302, -163.5354) -> (-144.0379, -176.0271) projected
  line L401 (-144.0379, -176.0271) -> (-134.5971, -176.0271) projected
  line L402 (-134.5971, -176.0271) -> (-134.5971, -164.0408) projected
  line L403 (-134.5971, -164.0408) -> (-83.7971, -164.0408) projected
  line L404 (-144.2491, -33.721) -> (-144.2491, -142.941) projected
  line L405 (-144.2491, -88.331) -> (-1.9844, -88.331) construction
  point P0 (0, 0)
  point P1 (-133.1068, -141.671)
  point P2 (-117.7089, -132.781)
  point P3 (-133.1068, -123.891)
  point P4 (-117.7089, -115.001)
  point P5 (-133.1068, -106.111)
  point P6 (-117.7089, -97.221)
  point P7 (-117.7089, -79.441)
  point P8 (-133.1068, -88.331)
  point P9 (-133.1068, -70.551)
  point P10 (-117.7089, -61.661)
  point P11 (-117.7089, -43.881)
  point P12 (-133.1068, -52.771)
  point P13 (-102.6268, -141.671)
  point P14 (-87.2289, -132.781)
  point P15 (-87.2289, -115.001)
  point P16 (-102.6268, -123.891)
  point P17 (-102.6268, -106.111)
  point P18 (-87.2289, -97.221)
  point P19 (-87.2289, -79.441)
  point P20 (-102.6268, -88.331)
  point P21 (-102.6268, -70.551)
  point P22 (-87.2289, -61.661)
  point P23 (-87.2289, -43.881)
  point P24 (-102.6268, -52.771)
  point P25 (-72.1468, -141.671)
  point P26 (-56.7489, -132.781)
  point P27 (-56.7489, -115.001)
  point P28 (-72.1468, -123.891)
  point P29 (-72.1468, -106.111)
  point P30 (-56.7489, -97.221)
  point P31 (-56.7489, -79.441)
  point P32 (-72.1468, -88.331)
  point P33 (-72.1468, -70.551)
  point P34 (-56.7489, -61.661)
  point P35 (-56.7489, -43.881)
  point P36 (-72.1468, -52.771)
  point P37 (-41.6668, -141.671)
  point P38 (-26.2689, -132.781)
  point P39 (-26.2689, -115.001)
  point P40 (-41.6668, -123.891)
  point P41 (-41.6668, -106.111)
  point P42 (-26.2689, -97.221)
  point P43 (-26.2689, -79.441)
  point P44 (-41.6668, -88.331)
  point P45 (-41.6668, -70.551)
  point P46 (-26.2689, -61.661)
  point P47 (-26.2689, -43.881)
  point P48 (-41.6668, -52.771)
  point P49 (-133.1068, -34.991)
  point P50 (-102.6268, -34.991)
  point P51 (-72.1468, -34.991)
  point P52 (-41.6668, -34.991)
  point P53 (-10.8709, -141.671)
  point P54 (-10.8709, -123.891)
  point P55 (-10.8709, -106.111)
  point P56 (-10.8709, -70.551)
  point P57 (-10.8709, -52.771)
  point P58 (-10.8709, -34.991)
  dimension "d150" = 12.7
  dimension "d151" = 12.7
  dimension "d152" = 12.7
  dimension "d153" = 12.7
  dimension "d154" = 5.08
  dimension "d155" = 5.08
  dimension "d156" = 5.08
  dimension "d158" = 5.08
  dimension "d159" = 5.08
  dimension "d162" = 35.56
  dimension "d165" = 30.48
  dimension "d168" = 3.81
  dimension "d169" = 12.7
  dimension "d170" = 12.7
  dimension "d171" = 30.48
  dimension "d174" = 12.7
  dimension "d175" = 12.7
  dimension "d187" = 12.7
  dimension "d188" = 12.7
  dimension "d189" = 12.7
  dimension "d191" = 12.7
  dimension "d192" = 12.7
  dimension "d193" = 12.7
  dimension "d195" = 5.08
  dimension "d196" = 5.08
  dimension "d199" = 5.08
  dimension "d205" = 46.99
  constraints: 698 end point, 20 horizontal alignment, 9 vertical alignment, 2 midpoint, 1 horizontal, 1 point on line, 1 vertical, 754 other
  measures "d150" distance between parallel lines of L5 L2
  measures "d151" distance between parallel lines of L11 L8
  measures "d152" distance between parallel lines of L17 L14
  measures "d153" distance between parallel lines of L23 L20
  measures "d154" distance between parallel lines of L1 L16
  measures "d155" distance between parallel lines of L2 L11
  measures "d156" distance between parallel lines of L23 L14
  measures "d158" distance between parallel lines of L7 L22
  measures "d159" distance between parallel lines of L15 L6
  measures "d162" distance of L8.end L52.start
  measures "d165" distance of L8.end L100.start
  measures "d168" distance from line of L33 L72.end
  measures "d169" distance between parallel lines of L321 L318
  measures "d170" distance between parallel lines of L327 L324
  measures "d171" distance of point (-133.107, -34.991) point (-102.627, -34.991)
  measures "d174" distance between parallel lines of L333 L330
  measures "d175" distance between parallel lines of L339 L336
  measures "d187" distance between parallel lines of L345 L342
  measures "d188" distance between parallel lines of L351 L348
  measures "d189" distance between parallel lines of L357 L354
  measures "d191" distance between parallel lines of L363 L360
  measures "d192" distance between parallel lines of L369 L366
  measures "d193" distance between parallel lines of L375 L372
  measures "d195" distance between parallel lines of L350 L341
  measures "d196" distance between parallel lines of L356 L347
  measures "d199" distance between parallel lines of L368 L359
  measures "d205" distance between parallel lines of L405 L320
extrude "Extrusion13" cut sketch "Sketch16" against normal through all contours L0 L1 L2 L3 L4 L5 | L6 L7 L8 L9 L10 L11 | L12 L13 L14 L15 L16 L17 | L18 L19 L20 L21 L22 L23 | L52 L63 L62 L64 L65 L54 | L53 L68 L67 L69 L60 L57 | L55 L58 L59 L61 L66 L56 | L70 L72 L74 L73 L71 L75 | L76 L87 L86 L88 L89 L78 | L77 L92 L91 L93 L84 L81 | L79 L82 L83 L85 L90 L80 | L94 L96 L98 L97 L95 L99 | L100 L111 L110 L112 L113 L102 | L101 L116 L115 L117 L108 L105 | L103 L106 L107 L109 L114 L104 | L118 L120 L122 L121 L119 L123 | L124 L135 L134 L136 L137 L126 | L125 L140 L139 L141 L132 L129 | L127 L130 L131 L133 L138 L128 | L142 L144 L146 L145 L143 L147 | L148 L159 L158 L160 L161 L150 | L149 L164 L163 L165 L156 L153 | L151 L154 L155 L157 L162 L152 | L166 L168 L170 L169 L167 L171 | L172 L183 L182 L184 L185 L174 | L173 L188 L187 L189 L180 L177 | L175 L178 L179 L181 L186 L176 | L190 L192 L194 L193 L191 L195 | L196 L207 L206 L208 L209 L198 | L197 L212 L211 L213 L204 L201 | L199 L202 L203 L205 L210 L200 | L214 L216 L218 L217 L215 L219 | L220 L231 L230 L232 L233 L222 | L221 L236 L235 L237 L228 L225 | L223 L226 L227 L229 L234 L224 | L238 L240 L242 L241 L239 L243 | L244 L255 L254 L256 L257 L246 | L245 L260 L259 L261 L252 L249 | L247 L250 L251 L253 L258 L248 | L262 L264 L266 L265 L263 L267 | L268 L279 L278 L280 L281 L270 | L269 L284 L283 L285 L276 L273 | L271 L274 L275 L277 L282 L272 | L286 L288 L290 L289 L287 L291 | L292 L303 L302 L304 L305 L294 | L293 L308 L307 L309 L300 L297 | L295 L298 L299 L301 L306 L296 | L310 L312 L314 L313 L311 L315 | L316 L317 L318 L319 L320 L321 | L322 L323 L324 L325 L326 L327 | L328 L329 L330 L331 L332 L333 | L334 L335 L336 L337 L338 L339 | L340 L341 L342 L343 L344 L345 | L346 L347 L348 L349 L350 L351 | L352 L353 L354 L355 L356 L357 | L358 L359 L360 L361 L362 L363 | L364 L365 L366 L367 L368 L369 | L370 L371 L372 L373 L374 L375